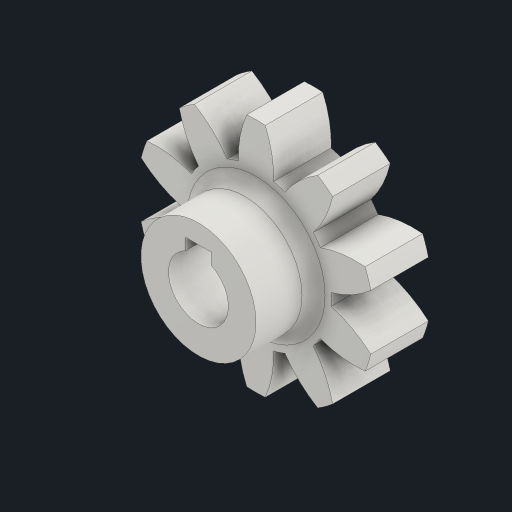
# Autodesk Inventor part: Spur Gear1
Saved by Autodesk Inventor 2024.3 (Build 283343000, 343)
## iProperties
CustomPartVersion: 1
Created: 2024-06-29
Part Number: Spur Gear1
Material: Steel
Document SubType Name: Modeling
Designer: Niler
Categories: <?xml version="1.0" encoding="UTF-16"?> <MemberInstance><Categories><FamilyTemplate><FamilyTemplateParameter ValueType="xs:double" Id="1" ObjectReferenceKey="da_z" ObjectType="kUserParameterObject"/><FamilyTemplateParameter ValueType="xs:double" Id="2" ObjectReferenceKey="da_b" ObjectType="kUserParameterObject"/><FamilyTemplateParameter ValueType="xs:double" Id="3" ObjectReferenceKey="da_beta" ObjectType="kUserParameterObject"/><FamilyTemplateParameter ValueType="xs:double" Id="4" ObjectReferenceKey="da_da" ObjectType="kUserParameterObject"/><FamilyTemplateParameter ValueType="xs:double" Id="5" ObjectReferenceKey="da_aw" ObjectType="kUserParameterObject"/><FamilyTemplateParameter ValueType="xs:string" Id="6" ObjectReferenceKey="EAIAABAAAACIAQAAAAAAAIAAAAAAAAAA" ObjectType="83910656" SubObjectId="SurfaceGeometry"/></FamilyTemplate><ParamToTemplateMap><ParamToTemplate CategoryParameter="//CategoryParameter[@InternalName='046C89C9-8512-4d59-83FE-43B91F4F132A']" TemplateParameter="1"/><ParamToTemplate CategoryParameter="//CategoryParameter[@InternalName='2552DF32-E462-4b46-AEBF-C6C7768E72AC']" TemplateParameter="2"/><ParamToTemplate CategoryParameter="//CategoryParameter[@InternalName='C9EE641D-15FC-4fae-A226-E94C4372FDD7']" TemplateParameter="3"/><ParamToTemplate><ParamToTemplate CategoryParameter="//CategoryParameter[@InternalName='00B6519A-459B-49c7-AD84-2E56D39A5744']" ConstantValue="0.000000"/></ParamToTemplate><ParamToTemplate><ParamToTemplate CategoryParameter="//CategoryParameter[@InternalName='04B31F0E-C7A6-4894-AA32-9629BEFACF47']" ConstantValue="1.000000"/></ParamToTemplate><ParamToTemplate><ParamToTemplate CategoryParameter="//CategoryParameter[@InternalName='43CBEC2E-7847-49e7-A936-2F7889FCB2D9']" ConstantValue="0.250000"/></ParamToTemplate><ParamToTemplate><ParamToTemplate CategoryParameter="//CategoryParameter[@InternalName='B1EFC894-105D-4ebd-86BF-FA20ED196853']" ConstantValue="0.350000"/></ParamToTemplate><ParamToTemplate><ParamToTemplate CategoryParameter="//CategoryParameter[@InternalName='51175063-3D10-4879-93E8-6246FE8B403D']" ConstantValue="2060000000.000000"/></ParamToTemplate><ParamToTemplate><ParamToTemplate CategoryParameter="//CategoryParameter[@InternalName='A3A52E27-4454-46a9-B0BD-C932399B70AF']" ConstantValue="0.300000"/></ParamToTemplate><ParamToTemplate><ParamToTemplate CategoryParameter="//CategoryParameter[@InternalName='91B76062-C214-41d9-B1B9-14D2AB99603D']" ConstantValue="0.350000"/></ParamToTemplate><ParamToTemplate><ParamToTemplate CategoryParameter="//CategoryParameter[@InternalName='374E806E-8B8A-4dda-A9AA-1039D6500AD2']" ConstantValue="2.857143"/></ParamToTemplate><ParamToTemplate><ParamToTemplate CategoryParameter="//CategoryParameter[@InternalName='2D373A89-B862-43d6-8D0B-0CBF12AB9F6C']" ConstantValue="0.349066"/></ParamToTemplate><ParamToTemplate CategoryParameter="//CategoryParameter[@InternalName='37777632-D6A2-4fac-9D53-DB8ACD95C989']" TemplateParameter="4"/><ParamToTemplate CategoryParameter="//CategoryParameter[@InternalName='FD1017F1-B727-4f7e-9707-0F86F1FF9423']" TemplateParameter="5"/><ParamToTemplate><ParamToTemplate CategoryParameter="//CategoryParameter[@InternalName='9E1B4470-B2D3-4ff1-B813-535BB4CDF51A']" ConstantValue="3520000.000000"/></ParamToTemplate><ParamToTemplate><ParamToTemplate CategoryParameter="//CategoryParameter[@InternalName='F8452263-BFF6-458c-9FB1-07C4B99E95CD']" ConstantValue="11400000.000000"/></ParamToTemplate><ParamToTemplate><ParamToTemplate CategoryParameter="//CategoryParameter[@InternalName='3E3BB259-FD49-497f-8171-6EBC954A3479']" ConstantValue="2.000000"/></ParamToTemplate><ParamToTemplate CategoryParameter="//CategoryParameter[@InternalName='27C3BAF2-7550-4e4b-AE2C-0DB134B7D9B7']" TemplateParameter="6"/></ParamToTemplateMap><Category DisplayName="Gear" InternalName="DC85795E-93AB-48d5-8EEE-5A27447B64BD" Mnemonic="Gear"><CategoryParameter DisplayName="z" InternalName="046C89C9-8512-4d59-83FE-43B91F4F132A" Mnemonic="z"/><CategoryParameter DisplayName="b" InternalName="2552DF32-E462-4b46-AEBF-C6C7768E72AC" Mnemonic="b"/><CategoryParameter DisplayName="||b|" InternalName="C9EE641D-15FC-4fae-A226-E94C4372FDD7" Mnemonic="beta"/><CategoryParameter DisplayName="x" InternalName="00B6519A-459B-49c7-AD84-2E56D39A5744" Mnemonic="x"/><CategoryParameter DisplayName="a*" InternalName="04B31F0E-C7A6-4894-AA32-9629BEFACF47" Mnemonic="a"/><CategoryParameter DisplayName="c*" InternalName="43CBEC2E-7847-49e7-A936-2F7889FCB2D9" Mnemonic="c"/><CategoryParameter DisplayName="r|.f|*" InternalName="B1EFC894-105D-4ebd-86BF-FA20ED196853" Mnemonic="rf"/><CategoryParameter DisplayName="E" InternalName="51175063-3D10-4879-93E8-6246FE8B403D" Mnemonic="E"/><CategoryParameter DisplayName="||m|" InternalName="A3A52E27-4454-46a9-B0BD-C932399B70AF" Mnemonic="mi"/><Category DisplayName="SpurGear" InternalName="26C5A22E-A91E-4dfd-A3B3-23CCAFAE1764" Mnemonic="SpurGear"><CategoryParameter DisplayName="m" InternalName="91B76062-C214-41d9-B1B9-14D2AB99603D" Mnemonic="m"/><CategoryParameter DisplayName="P" InternalName="374E806E-8B8A-4dda-A9AA-1039D6500AD2" Mnemonic="PP"/><CategoryParameter DisplayName="||a|" InternalName="2D373A89-B862-43d6-8D0B-0CBF12AB9F6C" Mnemonic="alpha"/><CategoryParameter DisplayName="d|.a|" InternalName="37777632-D6A2-4fac-9D53-DB8ACD95C989" Mnemonic="da"/><CategoryParameter DisplayName="a|.w|" InternalName="FD1017F1-B727-4f7e-9707-0F86F1FF9423" Mnemonic="aw"/><CategoryParameter DisplayName="||s||.Flim|" InternalName="9E1B4470-B2D3-4ff1-B813-535BB4CDF51A" Mnemonic="sFlim"/><CategoryParameter DisplayName="||s||.Hlim|" InternalName="F8452263-BFF6-458c-9FB1-07C4B99E95CD" Mnemonic="sHlim"/><CategoryParameter DisplayName="type" InternalName="3E3BB259-FD49-497f-8171-6EBC954A3479" Mnemonic="type"/><CategoryParameter DisplayName="PitchDiameter" InternalName="27C3BAF2-7550-4e4b-AE2C-0DB134B7D9B7" Mnemonic="IDS_PITCHDIAM"/></Category></Category></Categories></MemberInstance>
Density: 1 g/cm^3
Appearance: Steel
Author: Niler
Autodesk Inventor part; units mm, degrees
ref_plane "YZ Plane" through (0, 0, 0) normal (1, 0, 0) x (0, 1, 0)
ref_plane "XZ Plane" through (0, 0, 0) normal (0, 1, 0) x (-1, 0, 0)
ref_plane "XY Plane" through (0, 0, 0) normal (0, 0, 1) x (1, 0, 0)
sketch "Sketch1" plane through (0, 0, 0) normal (0, 0, 1) x (1, 0, 0)
  circle A0 centre (0, 0) radius 20.5216
  dimension "d0" = 41.0431
  constraints: 1 centre point
  measures "d0" diameter of A0
extrude "Extrusion1" add sketch "Sketch1" along normal blind 10
ref_plane "Work Plane2" through (0, 0, 5) normal (0, 0, 1) x (1, 0, 0)
sketch "Sketch2" plane through (0, 0, 0) normal (0, 0, -1) x (-1, 0, 0)
  circle A0 centre (0, 0) radius 20.5216 projected
  circle A1 centre (0, 0) radius 17.5
  dimension "d3" = 35
  constraints: 1 centre point, 1 coincident
  measures "d3" diameter of A1
surface extrude "Pitch Diameter" sketch "Sketch2" against normal through all shown no curves A1
ref_plane "Work Plane8" through (0, 0, 0) normal (0.9510565, 0.309017, 0) x (0, 0, 1)
ref_plane "Work Plane9" through (0, 0, 0) normal (1, 0, 0) x (0, 1, 0)
spur gear teeth "Spur Gear" teeth 10 pitch diameter 35 tip diameter 41.0431 root diameter 26.25 face width 10 start plane through (0, 0, 0) normal (0, 0, -1) x (-1, 0, 0)
sketch "Sketch3" plane through (0, 0, 10) normal (0, 0, 1) x (1, 0, 0)
  circle A0 centre (0, 0) radius 9
  circle A1 centre (0, 0) radius 5
  line L0 (-2, 0) -> (2, 0)
  line L1 (2, 0) -> (2, 6.5)
  line L2 (2, 6.5) -> (-2, 6.5)
  line L3 (-2, 6.5) -> (-2, 0)
  line L4 (2.2, 6.7) -> (2.2, -0.2)
  line L5 (2.2, -0.2) -> (-2.2, -0.2)
  line L6 (-2.2, -0.2) -> (-2.2, 6.7)
  line L7 (-2.2, 6.7) -> (2.2, 6.7)
  circle A2 centre (0, 0) radius 5.2
  point P0 (0, -5)
  point P1 (-2.2, 4.7117)
  point P2 (2.2, 4.7117)
  dimension "d50" = 10
  dimension "d49" = 18
  dimension "d52" = 11.5
  dimension "d53" = 4
  dimension "d54" = 0.2
  dimension "d55" = 0.2
  constraints: 16 end point, 4 parallel, 3 coincident, 2 centre point, 2 perpendicular, 2 vertical alignment, 1 horizontal, 1 midpoint, 5 other
  measures "d49" diameter of A0
  measures "d52" distance from line of point (0, -5) L2
  measures "d53" distance of L1.end L2.end
  measures "d54" distance between parallel lines of L1 L4
extrude "Extrusion2" cut sketch "Sketch3" against normal through all contours A1 L6 L5 L4 | A1 L4 A2 L6 | L4 L5 L6 A1 L3 L0 L1 | A1 L1 A2 L4 | L6 A2 L3 A1 | L1 L0 L3 A1 | A1 L3 A2 L1 | A2 L1 L2 L3 L6 L7 L4 | A2 L3 L2 L1
sketch "Sketch4" plane through (0, 0, 10) normal (0, 0, 1) x (1, 0, 0)
  line L0 (-2.2, 6.7) -> (2.2, 6.7) projected
  line L1 (2.2, 6.7) -> (2.2, 4.7117) projected
  arc A0 (-2.2, 4.7117) -> (2.2, 4.7117) centre (0, 0) ccw projected
  line L2 (-2.2, 4.7117) -> (-2.2, 6.7) projected
  arc A1 (-13.3277, 15.6047) -> (-9.9803, 8.524) centre (4.1841, 19.5517) ccw projected
  arc A2 (-9.9803, 8.524) -> (-11.1909, 6.8578) centre (0, 0) ccw projected
  arc A3 (-11.1909, 6.8578) -> (-18.9595, 7.8533) centre (-17.3018, -10.0211) ccw projected
  arc A4 (-18.9595, 7.8533) -> (-19.9546, 4.7907) centre (0, 0) ccw projected
  arc A5 (-19.9546, 4.7907) -> (-13.0845, 1.0298) centre (-8.1072, 18.277) ccw projected
  arc A6 (-13.0845, 1.0298) -> (-13.0845, -1.0298) centre (0, 0) ccw projected
  arc A7 (-13.0845, -1.0298) -> (-19.9546, -4.7907) centre (-8.1072, -18.277) ccw projected
  arc A8 (-19.9546, -4.7907) -> (-18.9595, -7.8533) centre (0, 0) ccw projected
  arc A9 (-18.9595, -7.8533) -> (-11.1909, -6.8578) centre (-17.3018, 10.0211) ccw projected
  arc A10 (-11.1909, -6.8578) -> (-9.9803, -8.524) centre (0, 0) ccw projected
  arc A11 (-9.9803, -8.524) -> (-13.3277, -15.6047) centre (4.1841, -19.5517) ccw projected
  arc A12 (-13.3277, -15.6047) -> (-10.7225, -17.4975) centre (0, 0) ccw projected
  arc A13 (-10.7225, -17.4975) -> (-5.0227, -12.1259) centre (-19.8877, -2.0625) ccw projected
  arc A14 (-5.0227, -12.1259) -> (-3.064, -12.7624) centre (0, 0) ccw projected
  arc A15 (-3.064, -12.7624) -> (-1.6101, -20.4583) centre (14.8772, -13.3583) ccw projected
  arc A16 (-1.6101, -20.4583) -> (1.6101, -20.4583) centre (0, 0) ccw projected
  arc A17 (1.6101, -20.4583) -> (3.064, -12.7624) centre (-14.8772, -13.3583) ccw projected
  arc A18 (3.064, -12.7624) -> (5.0227, -12.1259) centre (0, 0) ccw projected
  arc A19 (5.0227, -12.1259) -> (10.7225, -17.4975) centre (19.8877, -2.0625) ccw projected
  arc A20 (10.7225, -17.4975) -> (13.3277, -15.6047) centre (0, 0) ccw projected
  arc A21 (13.3277, -15.6047) -> (9.9803, -8.524) centre (-4.1841, -19.5517) ccw projected
  arc A22 (9.9803, -8.524) -> (11.1909, -6.8578) centre (0, 0) ccw projected
  arc A23 (11.1909, -6.8578) -> (18.9595, -7.8533) centre (17.3018, 10.0211) ccw projected
  arc A24 (18.9595, -7.8533) -> (19.9546, -4.7907) centre (0, 0) ccw projected
  arc A25 (19.9546, -4.7907) -> (13.0845, -1.0298) centre (8.1072, -18.277) ccw projected
  arc A26 (13.0845, -1.0298) -> (13.0845, 1.0298) centre (0, 0) ccw projected
  arc A27 (13.0845, 1.0298) -> (19.9546, 4.7907) centre (8.1072, 18.277) ccw projected
  arc A28 (19.9546, 4.7907) -> (18.9595, 7.8533) centre (0, 0) ccw projected
  arc A29 (18.9595, 7.8533) -> (11.1909, 6.8578) centre (17.3018, -10.0211) ccw projected
  arc A30 (11.1909, 6.8578) -> (9.9803, 8.524) centre (0, 0) ccw projected
  arc A31 (9.9803, 8.524) -> (13.3277, 15.6047) centre (-4.1841, 19.5517) ccw projected
  arc A32 (13.3277, 15.6047) -> (10.7225, 17.4975) centre (0, 0) ccw projected
  arc A33 (10.7225, 17.4975) -> (5.0227, 12.1259) centre (19.8877, 2.0625) ccw projected
  arc A34 (5.0227, 12.1259) -> (3.064, 12.7624) centre (0, 0) ccw projected
  arc A35 (3.064, 12.7624) -> (1.6101, 20.4583) centre (-14.8772, 13.3583) ccw projected
  arc A36 (1.6101, 20.4583) -> (-1.6101, 20.4583) centre (0, 0) ccw projected
  arc A37 (-1.6101, 20.4583) -> (-3.064, 12.7624) centre (14.8772, 13.3583) ccw projected
  arc A38 (-3.064, 12.7624) -> (-5.0227, 12.1259) centre (0, 0) ccw projected
  arc A39 (-5.0227, 12.1259) -> (-10.7225, 17.4975) centre (-19.8877, 2.0625) ccw projected
  arc A40 (-10.7225, 17.4975) -> (-13.3277, 15.6047) centre (0, 0) ccw projected
  circle A41 centre (0, 0) radius 10
  dimension "d58" = 20
  constraints: 1 centre point, 1 coincident
  measures "d58" diameter of A41
extrude "Extrusion3" add sketch "Sketch4" along normal blind 10 contours A41
fillet "Fillet1" radius 2 1 edges at (-10, 0, 10)
equation "\"d0\" = da_da"
equation "\"d1\" = da_b"
equation "\"d3\" = da_d"
equation "\"d16\" = da_aw"
equation "\"d43\" = da_aw"
equation "\"d46\" = da_aw"
equation "\"da_da\" = 41.043141"
equation "\"da_b\" = 10"
equation "\"da_d\" = 35"
equation "\"da_aw\" = 57"
body "Solid1"
body "Srf1"
